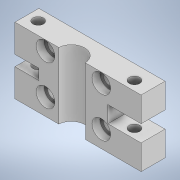
# Autodesk Inventor part: Podstawa
Saved by Autodesk Inventor 2021 (Build 250183000, 183)
## iProperties
Created: 2020-04-12
Part Number: Podstawa
Material: Ogólny
Document SubType Name: Modeling
Designer: dyrag
Density: 1 g/cm^3
Appearance: Domyślna
Author: dyrag
Autodesk Inventor part; units mm, degrees
ref_plane "YZ Plane" through (0, 0, 0) normal (1, 0, 0) x (0, 1, 0)
ref_plane "XZ Plane" through (0, 0, 0) normal (0, 1, 0) x (-1, 0, 0)
ref_plane "XY Plane" through (0, 0, 0) normal (0, 0, 1) x (1, 0, 0)
sketch "Szkic2" plane through (0, 0, 0) normal (0, 0, 1) x (1, 0, 0)
  line L0 (-44, 25) -> (51, 25)
  line L1 (-44, -25) -> (51, -25)
  line L2 (51, -25) -> (51, -6.25)
  line L3 (51, -6.25) -> (26, -6.25)
  line L4 (26, -6.25) -> (26, 6.25)
  line L5 (26, 6.25) -> (51, 6.25)
  line L6 (51, 6.25) -> (51, 25)
  line L7 (-44, -25) -> (-44, -4)
  line L8 (-44, -4) -> (-26, -4)
  line L9 (-26, -4) -> (-26, 4)
  line L10 (-26, 4) -> (-44, 4)
  line L11 (-44, 4) -> (-44, 25)
  line L12 (0, 35) -> (0, -35) projected
  line L13 (-63, 0) -> (70, 0) projected
  point P0 (0, 0)
  dimension "d7" = 95
  dimension "d8" = 25
  dimension "d9" = 12.5
  dimension "d10" = 18
  dimension "d11" = 50
  dimension "d12" = 8
  constraints: 24 end point, 8 perpendicular, 2 point on line, 2 vertical, 1 horizontal, 5 other
  measures "d7" distance of L1.end L1.start
  measures "d8" distance of L2.end L3.end
  measures "d9" distance of L3.end L4.end
  measures "d10" distance of L7.end L8.end
  measures "d11" distance of L1.start L0.start
  measures "d12" distance of L7.end L10.end
extrude "Wyciągnięcie proste1" add sketch "Szkic2" along normal blind 18
sketch "Szkic3" plane through (-44, -25, 0) normal (0, -1, 0) x (1, 0, 0)
  line L0 (0, 0) -> (95, 0) projected
  line L1 (95, 0) -> (95, 18) projected
  line L2 (0, 18) -> (95, 18) projected
  line L3 (0, 0) -> (0, 18) projected
  circle A0 centre (8, 8.5) radius 4
  circle A1 centre (83, 11) radius 4
  circle A2 centre (43, 18.5) radius 10
  point P0 (44, 0)
  dimension "d16" = 11
  dimension "d19" = 9.5
  dimension "d21" = 20
  dimension "d22" = 43
  dimension "d23" = 40
  dimension "d24" = 35
  dimension "d25" = 8
  dimension "d26" = 0.5
  dimension "d27" = 8
  constraints: 3 centre point
  measures "d16" vertical distance of A1.centre L0.end
  measures "d19" vertical distance of L2.start A0.centre
  measures "d21" diameter of A2
  measures "d22" horizontal distance of A2.centre L0.start
  measures "d23" horizontal distance of A1.centre A2.centre
  measures "d24" horizontal distance of A2.centre A0.centre
  measures "d25" diameter of A0
  measures "d26" distance from line of A2.centre L2
  measures "d27" diameter of A1
extrude "Wyciągnięcie proste2" cut sketch "Szkic3" against normal through all contours A2 L2 | L2 A2 | A0 | A1
sketch "Szkic4" plane through (0, 0, 18) normal (0, 0, 1) x (1, 0, 0)
  line L0 (0, 35) -> (0, -35) projected
  line L1 (-63, 0) -> (70, 0) projected
  point P0 (0, 0)
  point P1 (21, -12.3158)
  point P2 (21, 17.6842)
  point P3 (-21, 17.6842)
  point P4 (-21, -12.3158)
  dimension "d30" = 42
  dimension "d31" = 30
  constraints: 2 symmetric about line
  measures "d30" distance of point (-21, 17.684) point (21, 17.684)
  measures "d31" distance of point (21, 17.684) point (21, -12.316)
hole "Otwór1" at (21, -12.3158, 18) at (21, 17.6842, 18) at (-21, 17.6842, 18) at (-21, -12.3158, 18) direction (0, 0, -1) diameter 9 depth 20 tip angle 118 counterbore diameter 14 counterbore depth 6
